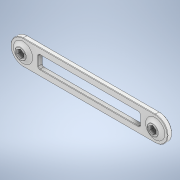
# Autodesk Inventor part: Long Bottom Nut Traps
Saved by Autodesk Inventor 2020 (Build 240168000, 168)
## iProperties
Created: 2020-06-20
Part Number: Long Bottom Nut Traps
Material: ABS Plastic
Document SubType Name: Modeling
Designer: Ishaan
Density: 1.06 g/cm^3
Appearance: Smooth - White
Author: Ishaan
Autodesk Inventor part; units mm, degrees
ref_plane "YZ Plane" through (0, 0, 0) normal (1, 0, 0) x (0, 1, 0)
ref_plane "XZ Plane" through (0, 0, 0) normal (0, 1, 0) x (-1, 0, 0)
ref_plane "XY Plane" through (0, 0, 0) normal (0, 0, 1) x (1, 0, 0)
sketch "Sketch1" plane through (0, 0, 0) normal (0, 0, 1) x (1, 0, 0)
  line L0 (88.5, -14) -> (-88.5, -14)
  line L1 (-88.5, -14) -> (-88.5, 14)
  line L2 (-88.5, 14) -> (88.5, 14)
  line L3 (88.5, 14) -> (88.5, -14)
  line L4 (88.5, -14) -> (-88.5, 14) construction
  line L5 (-88.5, -14) -> (88.5, 14) construction
  line L6 (-74.5, 0) -> (74.5, 0) construction
  line L7 (-60.5, -14) -> (-88.5, -14) construction
  line L8 (-88.5, -14) -> (-88.5, 14) construction
  line L9 (-88.5, 14) -> (-60.5, 14) construction
  line L10 (-60.5, 14) -> (-60.5, -14) construction
  line L11 (-60.5, -14) -> (-88.5, 14) construction
  line L12 (-88.5, -14) -> (-60.5, 14) construction
  point P0 (0, 0)
  point P1 (0, 0)
  dimension "d2" = 149
  dimension "d3" = 28
  constraints: 26 end point, 6 midpoint, 4 parallel, 3 horizontal, 3 perpendicular, 2 coincident
  measures "d2" distance of L6.start L6.end
  measures "d3" distance between parallel lines of L0 L2
extrude "Extrusion1" add sketch "Sketch1" along normal blind 5
sketch "Sketch2" plane through (0, 0, 5) normal (0, 0, 1) x (1, 0, 0)
  line L0 (88.5, 14) -> (-88.5, 14) projected
  line L1 (-88.5, 14) -> (-88.5, -14) projected
  line L2 (-88.5, -14) -> (88.5, -14) projected
  line L3 (88.5, -14) -> (88.5, 14) projected
  line L4 (-60.5, -14) -> (-88.5, -14) construction
  line L5 (-88.5, -14) -> (-88.5, 14) construction
  line L6 (-88.5, 14) -> (-60.5, 14) construction
  line L7 (-60.5, 14) -> (-60.5, -14) construction
  line L8 (-60.5, -14) -> (-88.5, 14) construction
  line L9 (-88.5, -14) -> (-60.5, 14) construction
  line L10 (-88.5, 14) -> (-88.5, -14) projected
  line L11 (57.5, -7) -> (-57.5, -7)
  line L12 (-57.5, -7) -> (-57.5, 7)
  line L13 (-57.5, 7) -> (57.5, 7)
  line L14 (57.5, 7) -> (57.5, -7)
  line L15 (57.5, -7) -> (-57.5, 7) construction
  line L16 (-57.5, -7) -> (57.5, 7) construction
  point P0 (0, 0)
  point P1 (-74.5, 0)
  dimension "d6" = 7
  dimension "d26" = 3
  constraints: 24 end point, 4 midpoint, 4 parallel, 3 collinear, 3 perpendicular, 2 horizontal
  measures "d6" distance between parallel lines of L0 L13
  measures "d26" distance between parallel lines of L12 L7
extrude "Extrusion2" cut sketch "Sketch2" against normal through all contours L11 L12 L13 L14
hole "Hole1" at (-74.5, 0, 0) at (74.5, 0, 0) direction (0, 0, 1) diameter 5.4 end through all
sketch "Sketch4" plane through (0, 0, 5) normal (0, 0, 1) x (1, 0, 0)
  circle A0 centre (-74.5, 0) radius 2.7 projected
  circle A1 centre (74.5, 0) radius 2.7 projected
  line L0 (-57.5, -7) -> (-57.5, 7) projected
  line L1 (-57.5, 7) -> (57.5, 7) projected
  line L2 (57.5, 7) -> (57.5, -7) projected
  line L3 (57.5, -7) -> (-57.5, -7) projected
  line L4 (88.5, 14) -> (-88.5, 14) projected
  line L5 (-88.5, 14) -> (-88.5, -14) projected
  line L6 (-88.5, -14) -> (88.5, -14) projected
  line L7 (88.5, -14) -> (88.5, 14) projected
  circle A2 centre (-74.5, 0) radius 2.7 projected
  line L8 (-74.5, 4.7631) -> (-70.375, 2.3816)
  line L9 (-70.375, 2.3816) -> (-70.375, -2.3816)
  line L10 (-70.375, -2.3816) -> (-74.5, -4.7631)
  line L11 (-74.5, -4.7631) -> (-78.625, -2.3816)
  line L12 (-78.625, -2.3816) -> (-78.625, 2.3816)
  line L13 (-78.625, 2.3816) -> (-74.5, 4.7631)
  line L14 (74.5, 4.7631) -> (78.625, 2.3816)
  line L15 (78.625, 2.3816) -> (78.625, -2.3816)
  line L16 (78.625, -2.3816) -> (74.5, -4.7631)
  line L17 (74.5, -4.7631) -> (70.375, -2.3816)
  line L18 (70.375, -2.3816) -> (70.375, 2.3816)
  line L19 (70.375, 2.3816) -> (74.5, 4.7631)
  circle A3 centre (-74.5, 0) radius 6.25
  circle A4 centre (74.5, 0) radius 2.7 projected
  circle A5 centre (74.5, 0) radius 6.25
  point P0 (0, 0)
  dimension "d19" = 8.25
  dimension "d20" = 12.5
  dimension "d21" = 12.5
  constraints: 24 end point, 4 coincident, 2 centre point, 2 vertical, 1 parallel, 26 other
  measures "d19" distance between parallel lines of L9 L12
  measures "d20" diameter of A3
  measures "d21" diameter of A5
extrude "Extrusion3" add sketch "Sketch4" along normal blind 3 contours A3 | A5
sketch "Sketch5" plane through (0, 0, 5) normal (0, 0, 1) x (1, 0, 0)
  circle A0 centre (-74.5, 0) radius 2.7 projected
  line L0 (-78.625, 2.3816) -> (-78.625, -2.3816) projected
  line L1 (-78.625, -2.3816) -> (-74.5, -4.7631) projected
  line L2 (-74.5, -4.7631) -> (-70.375, -2.3816) projected
  line L3 (-70.375, -2.3816) -> (-70.375, 2.3816) projected
  line L4 (-70.375, 2.3816) -> (-74.5, 4.7631) projected
  line L5 (-74.5, 4.7631) -> (-78.625, 2.3816) projected
  line L6 (70.375, 2.3816) -> (70.375, -2.3816) projected
  line L7 (70.375, -2.3816) -> (74.5, -4.7631) projected
  line L8 (74.5, -4.7631) -> (78.625, -2.3816) projected
  line L9 (78.625, -2.3816) -> (78.625, 2.3816) projected
  line L10 (78.625, 2.3816) -> (74.5, 4.7631) projected
  line L11 (74.5, 4.7631) -> (70.375, 2.3816) projected
  circle A1 centre (74.5, 0) radius 2.7 projected
  point P0 (0, 0)
extrude "Extrusion4" cut sketch "Sketch5" against normal blind 2
fillet "Fillet3" radius 5 2 edges at (68.25, 0, 5) (-80.75, 0, 5)
fillet "Fillet1" radius 2 4 edges at (-57.5, 7, 2.5) (-57.5, -7, 2.5) (57.5, 7, 2.5) (57.5, -7, 2.5)
fillet "Fillet2" radius 14 4 edges at (-88.5, 14, 2.5) (-88.5, -14, 2.5) (88.5, 14, 2.5) (88.5, -14, 2.5)
fillet "Fillet4" radius 0.5 28 edges at (-74.5, -2.7, 0) (-56.9142, -6.4142, 0) (0, -7, 0) (56.9142, -6.4142, 0) (57.5, 0, 0) (56.9142, 6.4142, 0) (0, 7, 0) (-56.9142, 6.4142, 0) (-57.5, 0, 0) (-56.9142, 6.4142, 5) (0, 7, 5) (56.9142, 6.4142, 5) (57.5, 0, 5) (56.9142, -6.4142, 5) (0, -7, 5) (-56.9142, -6.4142, 5) (-57.5, 0, 5) (84.3995, 9.8995, 0) (0, 14, 0) (-84.3995, 9.8995, 0) (0, -14, 0) (-84.3995, 9.8995, 5) (0, -14, 5) (84.3995, 9.8995, 5) (0, 14, 5) (74.5, -2.7, 0) (-80.75, 0, 8) (68.25, 0, 8)
body "Solid1"
